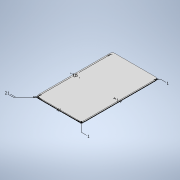
# Autodesk Inventor part: boden
Saved by Autodesk Inventor 2022 (Build 260153000, 153)
## iProperties
Created: 2022-04-04
Part Number: boden
Material: Generisch
Document SubType Name: Modeling
Designer: ga76xid
Density: 1 g/cm^3
Appearance: Vorgabe
Author: ga76xid
Autodesk Inventor part; units mm, degrees
ref_plane "YZ Plane" through (0, 0, 0) normal (1, 0, 0) x (0, 1, 0)
ref_plane "XZ Plane" through (0, 0, 0) normal (0, 1, 0) x (-1, 0, 0)
ref_plane "XY Plane" through (0, 0, 0) normal (0, 0, 1) x (1, 0, 0)
sketch "Skizze1" plane through (0, 0, 0) normal (0, 1, 0) x (-1, 0, 0)
  line L0 (1, 0) -> (40, 0)
  line L1 (41, 1) -> (41, 70)
  line L2 (40, 71) -> (1, 71)
  line L3 (0, 70) -> (0, 1)
  line L4 (42.5, 70.5) -> (42.5, 0.5)
  line L5 (40.5, -1.5) -> (0.5, -1.5)
  line L6 (-1.5, 0.5) -> (-1.5, 70.5)
  line L7 (0.5, 72.5) -> (40.5, 72.5)
  arc A0 (42.5, 70.5) -> (40.5, 72.5) centre (40.5, 70.5) ccw
  arc A1 (40.5, -1.5) -> (42.5, 0.5) centre (40.5, 0.5) ccw
  arc A2 (-1.5, 0.5) -> (0.5, -1.5) centre (0.5, 0.5) ccw
  arc A3 (0.5, 72.5) -> (-1.5, 70.5) centre (0.5, 70.5) ccw
  arc A4 (41, 70) -> (40, 71) centre (40, 70) ccw
  arc A5 (40, 0) -> (41, 1) centre (40, 1) ccw
  arc A6 (0, 1) -> (1, 0) centre (1, 1) ccw
  arc A7 (1, 71) -> (0, 70) centre (1, 70) ccw
  line L8 (1, 1) -> (1, 70)
  line L9 (1, 70) -> (40, 70)
  line L10 (40, 70) -> (40, 1)
  line L11 (40, 1) -> (1, 1)
  point P0 (0, 0)
  point P1 (41, 71)
  point P2 (41, 0)
  point P3 (0, 71)
  dimension "d0" = 41
  dimension "d1" = 71
  dimension "d2" = 1.5
  dimension "d3" = 2
  dimension "d4" = 1
  dimension "d5" = 1
  dimension "d6" = 1
  dimension "d9" = 1
  constraints: 24 end point, 16 point on circle, 16 tangent, 8 centre point, 8 point on line, 6 parallel, 4 equal radius, 3 perpendicular, 1 horizontal, 6 other
  measures "d0" distance of point (0, 71) point (41, 71)
  measures "d1" distance of point (41, 71) point (41, 0)
  measures "d2" distance between parallel lines of L1 L4
  measures "d3" radius of A0
  measures "d4" radius of A4
  measures "d5" radius of A6
  measures "d6" radius of A7
  measures "d9" distance between parallel lines of L3 L8
extrude "Extrusion1" add sketch "Skizze1" along normal blind 1 contours A6 L3 A7 L2 A4 L1 A5 L0 | L4 A1 L5 A2 L6 A3 L7 A0 | L8 L9 L10 L11
extrude "Extrusion2" add sketch "Skizze1" against normal blind 1 contours A6 L3 A7 L2 A4 L1 A5 L0
